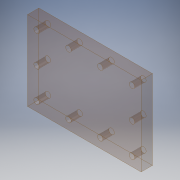
# Autodesk Inventor part: Acrylic Front
Saved by Autodesk Inventor 2018 (Build 220112000, 112)
## iProperties
Created: 2018-04-18
Part Number: Acrylic Front
Material: Polycarbonate, Smoke
Document SubType Name: Modeling
Designer: trent
Density: 1.2 g/cm^3
Appearance: Polycarbonate - Smoked
Author: trent
Autodesk Inventor part; units mm, degrees
ref_plane "YZ Plane" through (0, 0, 0) normal (1, 0, 0) x (0, 1, 0)
ref_plane "XZ Plane" through (0, 0, 0) normal (0, 1, 0) x (-1, 0, 0)
ref_plane "XY Plane" through (0, 0, 0) normal (0, 0, 1) x (1, 0, 0)
sketch "Sketch1" plane through (0, 0, 0) normal (0, 0, 1) x (1, 0, 0)
  line L0 (0, 0) -> (127, 0)
  line L1 (127, 0) -> (127, 88.9)
  line L2 (127, 88.9) -> (0, 88.9)
  line L3 (0, 88.9) -> (0, 0)
  circle A0 centre (10.16, 78.74) radius 3.0988
  circle A1 centre (10.16, 44.45) radius 3.0988
  circle A2 centre (10.16, 10.16) radius 3.0988
  circle A3 centre (45.72, 10.16) radius 3.0988
  circle A4 centre (116.84, 10.16) radius 3.0988
  circle A5 centre (116.84, 44.45) radius 3.0988
  circle A6 centre (116.84, 78.74) radius 3.0988
  circle A7 centre (45.72, 78.74) radius 3.0988
  circle A8 centre (81.28, 10.16) radius 3.0988
  circle A9 centre (81.28, 78.74) radius 3.0988
  dimension "d0" = 127
  dimension "d1" = 88.9
  dimension "d3" = 6.1976
  dimension "d4" = 10.16
  dimension "d5" = 10.16
  dimension "d6" = 10.16
  dimension "d7" = 10.16
  dimension "d8" = 44.45
  dimension "d10" = 10.16
  dimension "d11" = 10.16
  dimension "d12" = 10.16
  dimension "d13" = 10.16
  dimension "d14" = 44.45
  dimension "d15" = 10.16
  dimension "d16" = 10.16
  dimension "d17" = 10.16
  dimension "d18" = 10.16
  dimension "d42" = 35.56
  dimension "d43" = 35.56
  dimension "d44" = 35.56
  dimension "d46" = 35.56
  dimension "d47" = 35.56
  dimension "d49" = 35.56
  constraints: 10 centre point, 9 equal radius, 8 end point, 2 parallel, 1 horizontal, 1 perpendicular
  measures "d0" distance of L2.end L1.end
  measures "d1" distance of L1.end L0.end
  measures "d3" diameter of A0
  measures "d4" distance from line of L2 A0.centre
  measures "d5" distance from line of L3 A0.centre
  measures "d6" distance from line of L3 A2.centre
  measures "d7" distance from line of L0 A2.centre
  measures "d8" distance from line of L0 A1.centre
  measures "d10" distance from line of L2 A7.centre
  measures "d11" distance from line of L3 A1.centre
  measures "d12" distance from line of L2 A6.centre
  measures "d13" distance from line of L1 A6.centre
  measures "d14" distance from line of L0 A5.centre
  measures "d15" distance from line of L1 A5.centre
  measures "d16" distance from line of L0 A4.centre
  measures "d17" distance from line of L1 A4.centre
  measures "d18" distance from line of L0 A3.centre
  measures "d42" distance of A0.centre A7.centre
  measures "d43" distance of A7.centre A9.centre
  measures "d44" distance of A6.centre A9.centre
  measures "d46" distance of A8.centre A3.centre
  measures "d47" distance of A2.centre A3.centre
  measures "d49" distance of A4.centre A8.centre
extrude "Extrusion1" add sketch "Sketch1" along normal blind 12.7
equation "\"d6\" = d5"
equation "\"d7\" = d4"
equation "\"d8\" = 0.5 * d1"
equation "\"d10\" = d4"
equation "\"d11\" = d5"
equation "\"d12\" = d4"
equation "\"d13\" = d5"
equation "\"d14\" = 0.5 * d1"
equation "\"d15\" = d13"
equation "\"d16\" = d12"
equation "\"d17\" = d13"
equation "\"d18\" = d16"
equation "\"d43\" = d42"
equation "\"d44\" = d43"
equation "\"d46\" = d42"
equation "\"d47\" = d46"
equation "\"d49\" = d46"
body "Solid1"
